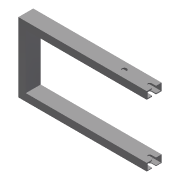
# Autodesk Inventor part: GARFO
Saved by Autodesk Inventor 2015 (Build 190159000, 159)
## iProperties
Created: 2016-08-09
Part Number: GARFO
Material: Aluminium AW-7020
Document SubType Name: Modeling
Designer: EriveltonDell
Density: 2.78 g/cm^3
Appearance: Stainless - Brushed
Mass: 1234.07 g
Surface Area: 731.335 cm^2
Volume: 443.911 cm^3
Author: EriveltonDell
Autodesk Inventor part; units mm, degrees
ref_plane "YZ Plane" through (0, 0, 0) normal (1, 0, 0) x (0, 1, 0)
ref_plane "XZ Plane" through (0, 0, 0) normal (0, 1, 0) x (-1, 0, 0)
ref_plane "XY Plane" through (0, 0, 0) normal (0, 0, 1) x (1, 0, 0)
sketch "Sketch1" plane through (0, 0, 0) normal (0, 1, 0) x (-1, 0, 0)
  line L0 (0, 0) -> (335, 0)
  line L1 (335, 0) -> (335, 167)
  line L2 (335, 167) -> (0, 167)
  dimension "d7" = 335
  dimension "d8" = 167
  dimension "d9" = 335
  constraints: 10 end point, 2 perpendicular, 1 horizontal
  measures "d7" distance of L0.start L0.end
  measures "d8" distance of L0.end L1.end
  measures "d9" distance of L1.end L2.end
sketch "Sketch2" plane through (0, 0, 0) normal (1, 0, 0) x (0, 1, 0)
  line L0 (0, 0) -> (-30, 0)
  line L1 (0, 0) -> (-20, 0)
  line L2 (-20, 0) -> (-20, -10)
  line L3 (-20, -10) -> (20, -10)
  line L4 (20, -10) -> (20, 10)
  line L5 (20, 10) -> (-20, 10)
  line L6 (-20, 10) -> (-20, 0)
  line L7 (17, 7) -> (17, -7)
  line L8 (17, -7) -> (-17, -7)
  line L9 (-17, -7) -> (-17, 0)
  line L10 (-17, 0) -> (-17, 7)
  line L11 (-17, 7) -> (17, 7)
  dimension "d20" = 20
  dimension "d21" = 10
  dimension "d22" = 40
  dimension "d23" = 20
  dimension "d24" = 40
  dimension "d25" = 3
  constraints: 24 end point, 5 perpendicular, 2 collinear, 2 point on line, 1 coincident, 1 horizontal, 4 other
  measures "d20" distance of L0.start L1.end
  measures "d21" distance of L1.end L2.end
  measures "d22" distance of L2.end L3.end
  measures "d23" distance of L3.end L4.end
  measures "d24" distance of L4.end L5.end
  measures "d25" distance between parallel lines of L4 L7
sweep "Sweep1" add profiles "Sketch2" path "Sketch1" contours L6 L5 L4 L3 L2 | L7 L8 L9 L10 L11
sketch "Sketch3" plane through (0, 0, 0) normal (0, 0, 1) x (1, 0, 0)
  line L0 (0, 0) -> (-12, 0)
  circle A0 centre (-12, 0) radius 5
  line L1 (-12, 5) -> (0, 5)
  line L2 (0, 5) -> (0, -5)
  line L3 (0, 20) -> (0, -20) projected
  line L4 (-12, -5) -> (0, -5.8056)
  dimension "d14" = 12
  dimension "d15" = 10
  constraints: 8 end point, 2 point on circle, 2 point on line, 1 centre point, 1 coincident, 1 horizontal, 1 parallel, 1 tangent
  measures "d14" distance of L0.start L0.end
  measures "d15" diameter of A0
extrude "Extrusion1" cut sketch "Sketch3" along normal through all both and the other way through all
shell "Shell1" thickness 2.5 removed faces 2 at (0, 10, 170.3333) at (0, -15.2685, 163.6667)
shell "Shell2" [suppressed]
hole "Hole1" at (-80, 0, 177) direction (0, 0, -1) diameter 13 depth 20 tip angle 118
sketch "Sketch6" plane through (0, -20, 177) normal (1, 0, 0) x (0, 0, -1)
  line L0 (169.5, 2.5) -> (185.1381, 2.5)
  line L1 (185.1381, 2.5) -> (185.1381, 38)
  line L2 (185.1381, 38) -> (169.5, 38)
  line L3 (169.5, 38) -> (169.5, 2.5)
  line L4 (184.5, 37.5) -> (2.5, 37.5) projected
  line L5 (2.5, 2.5) -> (17.4031, 2.5)
  line L6 (17.4031, 2.5) -> (17.4031, 37.5)
  line L7 (17.4031, 37.5) -> (2.5, 37.5)
  line L8 (2.5, 37.5) -> (2.5, 2.5)
  point P0 (177, 20)
  constraints: 16 end point, 4 parallel, 2 horizontal, 2 perpendicular, 1 point on line
extrude "Extrusion2" cut sketch "Sketch6" against normal blind 20
body "Solid1"
